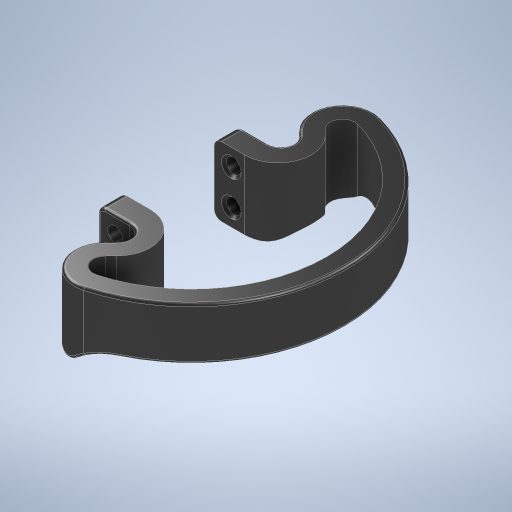
# Autodesk Inventor part: ShoulderBumper
Saved by Autodesk Inventor 2024.2 (Build 282272000, 272)
## iProperties
Created: 2024-01-20
Part Number: ShoulderBumper
Material: ABS Plastic
Document SubType Name: Modeling
Designer: Masato Kubotera
Density: 1.06 g/cm^3
Appearance: Glossy - Black
Mass: 50.6919 g
Surface Area: 172.591 cm^2
Volume: 47.8225 cm^3
Catalog Web Link: https://www.poly-maker.jp/polyflex-tpu90.html
Author: Masato Kubotera
Autodesk Inventor part; units mm, degrees
ref_plane "YZ Plane" through (0, 0, 0) normal (1, 0, 0) x (0, 1, 0)
ref_plane "XZ Plane" through (0, 0, 0) normal (0, 1, 0) x (-1, 0, 0)
ref_plane "XY Plane" through (0, 0, 0) normal (0, 0, 1) x (1, 0, 0)
sketch "Sketch1" plane through (0, 0, 0) normal (0, 0, 1) x (1, 0, 0)
  arc A0 (60.49, 26.5485) -> (-60.49, 26.5485) centre (0, 10) ccw
  line L0 (-28.25, 0) -> (-28.25, 13)
  line L1 (-19.25, 0) -> (-19.25, 12.3787)
  line L2 (-37.2694, 16.736) -> (-39.5942, 14.4112)
  line L3 (-28.25, 7) -> (14.3863, 7) construction
  line L4 (-28.25, 0) -> (-19.25, 0)
  line L5 (-19.25, 0) -> (19.25, 0) construction
  line L6 (0, 0) -> (0, 72.7128)
  line L7 (-28.25, 1) -> (-29.25, 1) construction
  line L8 (-29.25, 1) -> (-29.25, 13) construction
  line L9 (-29.25, 13) -> (-28.25, 13) construction
  line L10 (-29.25, 4.25) -> (-32.25, 4.25) construction
  line L11 (-32.25, 4.25) -> (-32.25, 9.75) construction
  line L12 (-32.25, 9.75) -> (-29.25, 9.75) construction
  line L13 (-40, 58.3) -> (40, 58.3) construction
  line L14 (-42.5727, 22.0393) -> (-44.8975, 19.7145)
  line L15 (28.25, 23.1131) -> (28.25, 23.1131)
  line L16 (19.25, 46.2552) -> (19.25, 46.2552)
  arc A1 (53.2558, 24.5694) -> (-53.2558, 24.5694) centre (0, 10) ccw
  arc A2 (-28.25, 13) -> (-37.2694, 16.736) centre (-33.5334, 13) ccw
  arc A3 (-53.2558, 24.5694) -> (-44.8975, 19.7145) centre (-48.433, 23.25) ccw
  arc A4 (-19.25, 12.3787) -> (-42.5727, 22.0393) centre (-32.9121, 12.3787) ccw
  line L17 (28.25, 0) -> (28.25, 13)
  line L18 (19.25, 0) -> (19.25, 12.3787)
  line L19 (28.25, 0) -> (19.25, 0)
  line L20 (42.5727, 22.0393) -> (44.8975, 19.7145)
  arc A5 (39.5942, 14.4112) -> (60.49, 26.5485) centre (48.433, 23.25) ccw
  arc A6 (37.2694, 16.736) -> (28.25, 13) centre (33.5334, 13) ccw
  arc A7 (44.8975, 19.7145) -> (53.2558, 24.5694) centre (48.433, 23.25) ccw
  arc A8 (42.5727, 22.0393) -> (19.25, 12.3787) centre (32.9121, 12.3787) ccw
  line L21 (37.2694, 16.736) -> (39.5942, 14.4112)
  line L22 (-37.2694, 16.736) -> (-42.5727, 22.0393) construction
  arc A9 (-60.49, 26.5485) -> (-39.5942, 14.4112) centre (-48.433, 23.25) ccw
  point P0 (62.5907, 15.3821)
  point P1 (0, 65.2128)
  dimension "d1" = 125.4255
  dimension "d2" = 10
  dimension "d3" = 12
  dimension "d4" = 1
  dimension "d5" = 5.5
  dimension "d6" = 3
  dimension "d7" = 1
  dimension "d8" = 9
  dimension "d9" = 38.5
  dimension "d12" = 51.3
  dimension "d13" = 14.4128
  dimension "d15" = 7.5
  dimension "d16" = 7.5
  dimension "d17" = 45
  dimension "d26" = 14
  dimension "d42" = 5
  dimension "d46" = 1
  dimension "d47" = 80
  constraints: 46 end point, 23 point on circle, 12 symmetric about line, 10 centre point, 7 horizontal, 7 tangent, 5 point on line, 5 vertical, 3 coincident, 1 collinear, 1 midpoint, 1 parallel, 1 perpendicular, 6 other
  measures "d1" diameter of A0
  measures "d2" distance of point (0, 0) A0.centre
  measures "d3" diameter of L7 L3
  measures "d4" distance between parallel lines of L4 L7
  measures "d5" diameter of L10 L3
  measures "d6" distance of L11.end L12.end
  measures "d7" distance of L0.end L8.end
  measures "d8" distance between parallel lines of L1 L0
  measures "d9" diameter of L1 L6
  measures "d12" distance between parallel lines of L13 L3
  measures "d13" distance from line of L6.end L13
  measures "d15" distance between parallel lines of L2 L14
  measures "d16" radial gap between concentric circles of A0 A1
  measures "d17" angle of L0 L2
  measures "d26" diameter of L4 L3
  measures "d42" radius of A3
  measures "d46" distance edge to line of A9 L12
  measures "d47" distance of L13.start L13.end
extrude "Extrusion1" add sketch "Sketch1" against normal blind 28.25 contours L6 A1 A3 L14 A4 L1 L4 L0 A2 L2 A9 A0
sketch "Sketch2" plane through (-28.25, 0, 0) normal (-1, 0, 0) x (0, 0, 1)
  line L0 (0, 7) -> (-28.25, 7) construction
  line L1 (-28.25, 12.3787) -> (-28.25, 0) projected
  circle A0 centre (-7, 7) radius 6 construction
  circle A1 centre (-21.25, 7) radius 6 construction
  line L2 (0, 0) -> (-28.25, 0) projected
  line L3 (-14.125, 0) -> (-14.125, 7) construction
  line L4 (0, 13) -> (0, 0) projected
  circle A2 centre (-7, 7) radius 3.05
  circle A3 centre (-21.25, 7) radius 3.05
  point P0 (0, 7)
  point P1 (-28.5, 51.788)
  dimension "d20" = 12
  dimension "d22" = 1
  dimension "d23" = 6.1
  dimension "d39" = 28.25
  dimension "d40" = 14.25
  constraints: 4 centre point, 4 end point, 2 coincident, 2 midpoint, 2 point on line, 1 equal radius, 1 horizontal, 3 other
  measures "d20" diameter of A0
  measures "d22" distance edge to line of A0 L4
  measures "d23" diameter of A2
  measures "d39" distance of L2.start L2.end
  measures "d40" distance of A1.centre A0.centre
extrude "Extrusion2" cut sketch "Sketch2" against normal up to surface (9 mm away)
fillet "Fillet1" radius 3 2 edges at (-23.75, 0, 0) (-23.75, 0, -28.25)
sketch "Sketch3" plane through (0, 65.2128, 0) normal (1, 0, 0) x (0, 0, -1)
  line L0 (0, 7.5) -> (28.25, 7.5) projected
  line L1 (21.25, 7.5) -> (21.25, -28.2128)
  arc A0 (21.25, -28.2128) -> (28.25, -43.4114) centre (41.25, -28.2128) ccw
  line L2 (28.25, -52.8341) -> (28.25, -62.2128) projected
  circle A1 centre (41.25, -28.2128) radius 18 construction
  circle A2 centre (41.25, -39.2128) radius 7 construction
  line L3 (41.25, -28.2128) -> (41.25, -46.2128) construction
  circle A3 centre (21.25, -58.2128) radius 3.05 projected
  line L4 (28.25, -43.4114) -> (28.25, 7.5)
  point P0 (0, -65.2128)
  point P1 (28.25, -25.8725)
  dimension "d30" = 36
  dimension "d31" = 14
  dimension "d32" = 20
  dimension "d33" = 19
  dimension "d34" = 2
  constraints: 6 end point, 3 point on line, 2 centre point, 2 point on circle, 2 vertical, 1 coincident, 1 collinear, 1 tangent, 1 vertical alignment, 3 other
  measures "d31" diameter of A2
  measures "d32" horizontal distance of A2.centre A3.centre
  measures "d33" vertical distance of A2.centre A3.centre
extrude "Extrusion3" cut sketch "Sketch3" against normal through all contours L0 L4 A0 L1
mirror "Mirror1" about plane through (0, 72.7128, 0) normal (1, 0, 0)
fillet "Fillet2" radius 10 4 edges at (32.915, 21.8013, -28.25) (57.0337, 21.8013, -28.25) (-32.915, 21.8013, -28.25) (-57.0337, 21.8013, -28.25)
fillet "Fillet3" radius 1 24 edges at (-58.8739, 31.6045, -21.9915) (-38.4318, 15.5736, -28.25) (-36.6109, 17.2947, -28.25) (-29.0468, 15.7901, -28.25) (-28.25, 8, -28.25) (-28.25, 0.8787, -27.3713) (-28.25, 0, -14.125) (-28.25, 0.8787, -0.8787) (-28.25, 8, 0) (-31.5116, 17.8813, 0) (-38.4318, 15.5736, 0) (0, 72.7128, 0) (38.4318, 15.5736, 0) (31.5116, 17.8813, 0) (28.25, 8, 0) (28.25, 0.8787, -0.8787) (28.25, 0, -14.125) (28.25, 0.8787, -27.3713) (28.25, 8, -28.25) (36.6109, 17.2947, -28.25) (29.0468, 15.7901, -28.25) (38.4318, 15.5736, -28.25) (58.8739, 31.6045, -21.9915) (0, 72.7128, -21.25)
chamfer "Chamfer1" distance 1 angle 45 4 edges at (-19.25, 7, -10.05) (-19.25, 7, -24.3) (19.25, 7, -10.05) (19.25, 7, -24.3)
body "Solid1"
